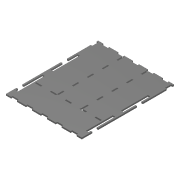
# Autodesk Inventor part: base
Saved by Autodesk Inventor 2020 (Build 240168000, 168)
## iProperties
Created: 2021-09-21
Part Number: base
Material: Generic
Document SubType Name: Modeling
Designer: pablo
Density: 1 g/cm^3
Appearance: Smooth - Black
Mass: 365.55 g
Surface Area: 1587.23 cm^2
Volume: 365.55 cm^3
Author: pablo
Autodesk Inventor part; units mm, degrees
ref_plane "YZ Plane" through (0, 0, 0) normal (1, 0, 0) x (0, 1, 0)
ref_plane "XZ Plane" through (0, 0, 0) normal (0, 1, 0) x (-1, 0, 0)
ref_plane "XY Plane" through (0, 0, 0) normal (0, 0, 1) x (1, 0, 0)
sketch "Sketch1" plane through (0, 0, 0) normal (0, 1, 0) x (-1, 0, 0)
  line L0 (127.5, -155) -> (-127.5, -155)
  line L1 (-127.5, -155) -> (-127.5, 155)
  line L2 (-127.5, 155) -> (127.5, 155)
  line L3 (127.5, 155) -> (127.5, -155)
  line L4 (127.5, -155) -> (-127.5, 155) construction
  line L5 (-127.5, -155) -> (127.5, 155) construction
  point P0 (0, 0)
  dimension "d0" = 255
  dimension "d1" = 310
  constraints: 12 end point, 2 midpoint, 2 parallel, 1 horizontal, 1 perpendicular
  measures "d0" distance of L1.end L2.end
  measures "d1" distance of L0.end L1.end
extrude "base" add sketch "Sketch1" along normal blind 5
sketch "Sketch3" plane through (0, 5, 0) normal (0, 1, 0) x (1, 0, 0)
  line L0 (127.5, 155) -> (-127.5, 155)
  line L1 (-127.5, 155) -> (-127.5, -155)
  line L2 (-127.5, 150) -> (-122.5, 150)
  line L3 (-122.5, 150) -> (-122.5, 130)
  line L4 (-122.5, 130) -> (-127.5, 130)
  line L5 (-127.5, 130) -> (-127.5, 150)
  line L6 (-127.5, 100) -> (-122.5, 100)
  line L7 (-122.5, 100) -> (-122.5, 80)
  line L8 (-122.5, 80) -> (-127.5, 80)
  line L9 (-127.5, 80) -> (-127.5, 100)
  line L10 (-127.5, 50) -> (-122.5, 50)
  line L11 (-122.5, 50) -> (-122.5, 30)
  line L12 (-122.5, 30) -> (-127.5, 30)
  line L13 (-127.5, 30) -> (-127.5, 50)
  line L14 (-127.5, 0) -> (-122.5, 0)
  line L15 (-122.5, 0) -> (-122.5, -20)
  line L16 (-122.5, -20) -> (-127.5, -20)
  line L17 (-127.5, -20) -> (-127.5, 0)
  line L18 (-127.5, -50) -> (-122.5, -50)
  line L19 (-122.5, -50) -> (-122.5, -70)
  line L20 (-122.5, -70) -> (-127.5, -70)
  line L21 (-127.5, -70) -> (-127.5, -50)
  line L22 (-127.5, -100) -> (-122.5, -100)
  line L23 (-122.5, -100) -> (-122.5, -120)
  line L24 (-122.5, -120) -> (-127.5, -120)
  line L25 (-127.5, -120) -> (-127.5, -100)
  line L26 (122.5, 50) -> (127.5, 50)
  line L27 (127.5, 30) -> (122.5, 30)
  line L28 (127.5, 50) -> (127.5, 30)
  line L29 (122.5, 30) -> (122.5, 50)
  line L30 (122.5, 0) -> (127.5, 0)
  line L31 (127.5, 0) -> (127.5, -20)
  line L32 (127.5, -20) -> (122.5, -20)
  line L33 (122.5, -20) -> (122.5, 0)
  line L34 (122.5, -50) -> (127.5, -50)
  line L35 (127.5, -50) -> (127.5, -70)
  line L36 (127.5, -70) -> (122.5, -70)
  line L37 (122.5, -70) -> (122.5, -50)
  line L38 (122.5, -100) -> (127.5, -100)
  line L39 (127.5, -100) -> (127.5, -120)
  line L40 (127.5, -120) -> (122.5, -120)
  line L41 (122.5, -120) -> (122.5, -100)
  line L42 (127.5, 80) -> (122.5, 80)
  line L43 (127.5, 100) -> (127.5, 80)
  line L44 (122.5, 80) -> (122.5, 100)
  line L45 (122.5, 100) -> (127.5, 100)
  line L46 (127.5, 130) -> (122.5, 130)
  line L47 (127.5, 150) -> (127.5, 130)
  line L48 (122.5, 130) -> (122.5, 150)
  line L49 (122.5, 150) -> (127.5, 150)
  point P0 (0, 0)
  point P1 (-127.5, 105)
  point P2 (-127.5, 55)
  point P3 (-127.5, 5)
  point P4 (-127.5, -45)
  point P5 (-127.5, -95)
  point P6 (122.5, 155)
  point P7 (122.5, 55)
  point P8 (122.5, 5)
  point P9 (122.5, -95)
  point P10 (122.5, -45)
  point P11 (122.5, 105)
  dimension "d4" = 5
  dimension "d5" = 20
  dimension "d8" = 50
  dimension "d15" = 250
  constraints: 100 end point, 1 horizontal, 1 point on line, 1 vertical, 99 other
  measures "d4" distance of L3.end L4.end
  measures "d5" distance of L2.end L3.end
  measures "d8" distance of L0.end point (-127.5, 105)
  measures "d15" distance of L0.end point (122.5, 155)
extrude "Encaixe Laterais" cut sketch "Sketch3" against normal blind 5 contours L2 L3 L4 L1 | L22 L23 L24 L1 | L10 L11 L12 L1 | L26 L28 L27 L29 | L38 L39 L40 L41 | L46 L48 L49 L47
sketch "Sketch4" plane through (0, 5, 0) normal (0, 1, 0) x (1, 0, 0)
  line L0 (-127.5, 150) -> (-122.5, 150) projected
  line L1 (122.5, 150) -> (127.5, 150) projected
  line L2 (-122.5, 150) -> (122.5, 150)
  line L3 (-40.8333, 150) -> (-35.8333, 150)
  line L4 (-35.8333, 150) -> (-35.8333, 130)
  line L5 (-35.8333, 130) -> (-40.8333, 130)
  line L6 (-40.8333, 130) -> (-40.8333, 150)
  line L7 (40.8333, 150) -> (45.8333, 150)
  line L8 (45.8333, 150) -> (45.8333, 130)
  line L9 (45.8333, 130) -> (40.8333, 130)
  line L10 (40.8333, 130) -> (40.8333, 150)
  line L11 (-40.8333, 100) -> (-35.8333, 100)
  line L12 (-35.8333, 100) -> (-35.8333, 80)
  line L13 (-35.8333, 80) -> (-40.8333, 80)
  line L14 (-40.8333, 80) -> (-40.8333, 100)
  line L15 (40.8333, 100) -> (45.8333, 100)
  line L16 (45.8333, 100) -> (45.8333, 80)
  line L17 (45.8333, 80) -> (40.8333, 80)
  line L18 (40.8333, 80) -> (40.8333, 100)
  line L19 (-40.8333, 50) -> (-35.8333, 50)
  line L20 (-35.8333, 50) -> (-35.8333, 30)
  line L21 (-35.8333, 30) -> (-40.8333, 30)
  line L22 (-40.8333, 30) -> (-40.8333, 50)
  line L23 (40.8333, 50) -> (45.8333, 50)
  line L24 (45.8333, 50) -> (45.8333, 30)
  line L25 (45.8333, 30) -> (40.8333, 30)
  line L26 (40.8333, 30) -> (40.8333, 50)
  line L27 (-40.8333, 0) -> (-35.8333, 0)
  line L28 (-35.8333, 0) -> (-35.8333, -20)
  line L29 (-35.8333, -20) -> (-40.8333, -20)
  line L30 (-40.8333, -20) -> (-40.8333, 0)
  line L31 (40.8333, 0) -> (45.8333, 0)
  line L32 (45.8333, 0) -> (45.8333, -20)
  line L33 (45.8333, -20) -> (40.8333, -20)
  line L34 (40.8333, -20) -> (40.8333, 0)
  line L35 (-40.8333, -50) -> (-35.8333, -50)
  line L36 (-35.8333, -50) -> (-35.8333, -70)
  line L37 (-35.8333, -70) -> (-40.8333, -70)
  line L38 (-40.8333, -70) -> (-40.8333, -50)
  line L39 (40.8333, -50) -> (45.8333, -50)
  line L40 (45.8333, -50) -> (45.8333, -70)
  line L41 (45.8333, -70) -> (40.8333, -70)
  line L42 (40.8333, -70) -> (40.8333, -50)
  point P0 (0, 0)
  dimension "d22" = 245
  dimension "d23" = 5
  dimension "d24" = 20
  dimension "d25" = 81.6667
  dimension "d28" = 81.6667
  dimension "d31" = 50
  constraints: 82 end point, 3 horizontal, 2 collinear, 2 parallel, 1 perpendicular, 1 point on line, 1 vertical, 70 other
  measures "d22" distance of L0.end L1.start
  measures "d23" distance of L4.end L5.end
  measures "d24" distance of L3.end L4.end
  measures "d25" distance of L0.end L3.start
  measures "d28" distance of L3.start L7.start
  measures "d31" distance of L3.start L11.start
extrude "Encaixe Divisórias 22cm" cut sketch "Sketch4" against normal blind 5
sketch "Sketch5" plane through (0, 5, 0) normal (0, 1, 0) x (1, 0, 0)
  line L0 (-127.5, -155) -> (127.5, -155) projected
  line L1 (-110, -155) -> (-90, -155)
  line L2 (-90, -155) -> (-90, -150)
  line L3 (-90, -150) -> (-110, -150)
  line L4 (-110, -150) -> (-110, -155)
  line L5 (-60, -155) -> (-40, -155)
  line L6 (-40, -155) -> (-40, -150)
  line L7 (-40, -150) -> (-60, -150)
  line L8 (-60, -150) -> (-60, -155)
  line L9 (-10, -155) -> (10, -155)
  line L10 (10, -155) -> (10, -150)
  line L11 (10, -150) -> (-10, -150)
  line L12 (-10, -150) -> (-10, -155)
  line L13 (40, -155) -> (60, -155)
  line L14 (60, -155) -> (60, -150)
  line L15 (60, -150) -> (40, -150)
  line L16 (40, -150) -> (40, -155)
  line L17 (90, -155) -> (110, -155)
  line L18 (110, -155) -> (110, -150)
  line L19 (110, -150) -> (90, -150)
  line L20 (90, -150) -> (90, -155)
  line L21 (-110, 155) -> (-110, 150)
  line L22 (-90, 155) -> (-110, 155)
  line L23 (-110, 150) -> (-90, 150)
  line L24 (-90, 150) -> (-90, 155)
  line L25 (-60, 155) -> (-60, 150)
  line L26 (-40, 155) -> (-60, 155)
  line L27 (-40, 150) -> (-40, 155)
  line L28 (-10, 155) -> (-10, 150)
  line L29 (10, 155) -> (-10, 155)
  line L30 (10, 150) -> (10, 155)
  line L31 (-10, 150) -> (10, 150)
  line L32 (-60, 150) -> (-40, 150)
  line L33 (40, 155) -> (40, 150)
  line L34 (40, 150) -> (60, 150)
  line L35 (60, 155) -> (40, 155)
  line L36 (60, 150) -> (60, 155)
  line L37 (90, 155) -> (90, 150)
  line L38 (90, 150) -> (110, 150)
  line L39 (110, 155) -> (90, 155)
  line L40 (110, 150) -> (110, 155)
  point P0 (0, 0)
  dimension "d36" = 20
  dimension "d37" = 5
  dimension "d40" = 50
  dimension "d45" = 17.5
  dimension "d46" = 17.5
  dimension "d49" = 305
  constraints: 80 end point, 2 horizontal, 2 parallel, 1 collinear, 1 perpendicular, 1 point on line, 1 vertical, 71 other
  measures "d36" distance of L3.end L2.end
  measures "d37" distance of L2.end L1.end
  measures "d40" distance of L1.start L5.start
  measures "d45" distance of L0.start L1.start
  measures "d46" distance of L17.end L0.end
  measures "d49" distance of L1.start L21.end
extrude "Extrusion4" cut sketch "Sketch5" against normal blind 5
sketch "Sketch6" plane through (0, 5, 0) normal (0, 1, 0) x (1, 0, 0)
  line L0 (-110, -155) -> (-110, -150) projected
  line L1 (110, -150) -> (110, -155) projected
  line L2 (-35.8333, -70) -> (-40.8333, -70) projected
  line L3 (-110, -70) -> (-90, -70)
  line L4 (-90, -70) -> (-90, -75)
  line L5 (-90, -75) -> (-110, -75)
  line L6 (-110, -75) -> (-110, -70)
  line L7 (-60, -70) -> (-40, -70)
  line L8 (-40, -70) -> (-40, -75)
  line L9 (-40, -75) -> (-60, -75)
  line L10 (-60, -75) -> (-60, -70)
  line L11 (-10, -70) -> (10, -70)
  line L12 (10, -70) -> (10, -75)
  line L13 (10, -75) -> (-10, -75)
  line L14 (-10, -75) -> (-10, -70)
  line L15 (40, -70) -> (60, -70)
  line L16 (60, -70) -> (60, -75)
  line L17 (60, -75) -> (40, -75)
  line L18 (40, -75) -> (40, -70)
  line L19 (90, -70) -> (110, -70)
  line L20 (110, -70) -> (110, -75)
  line L21 (110, -75) -> (90, -75)
  line L22 (90, -75) -> (90, -70)
  point P0 (0, 0)
  dimension "d56" = 20
  dimension "d57" = 5
  dimension "d60" = 50
  constraints: 40 end point, 2 horizontal, 2 parallel, 1 collinear, 1 perpendicular, 31 other
  measures "d56" distance of L4.end L5.end
  measures "d57" distance of L3.end L4.end
  measures "d60" distance of L3.start L7.start
extrude "Extrusion5" cut sketch "Sketch6" against normal blind 5
sketch "Sketch7" plane through (0, 5, 0) normal (0, 1, 0) x (1, 0, 0)
  line L0 (-127.5, -155) -> (-110, -155) projected
  line L1 (-90, -155) -> (-60, -155) projected
  line L2 (-114.5, -10) -> (-122.5, -10)
  line L3 (-122.5, -10) -> (-122.5, 80)
  line L4 (-122.5, 80) -> (-114.5, 80)
  line L5 (-114.5, 80) -> (-114.5, -10)
  line L6 (-114.5, -10) -> (-122.5, 80) construction
  line L7 (-122.5, -10) -> (-114.5, 80) construction
  line L8 (-127.5, 155) -> (-127.5, 150) projected
  line L9 (-122.5, -128) -> (-114.5, -128)
  line L10 (-114.5, -128) -> (-114.5, -38)
  line L11 (-114.5, -38) -> (-122.5, -38)
  line L12 (-122.5, -38) -> (-122.5, -128)
  line L13 (-122.5, -128) -> (-114.5, -38) construction
  line L14 (-114.5, -128) -> (-122.5, -38) construction
  line L15 (0, -20) -> (0, -40)
  line L16 (114.5, -10) -> (122.5, -10)
  line L17 (122.5, -10) -> (122.5, 80)
  line L18 (122.5, 80) -> (114.5, 80)
  line L19 (114.5, 80) -> (114.5, -10)
  line L20 (114.5, -10) -> (122.5, 80) construction
  line L21 (122.5, -10) -> (114.5, 80) construction
  line L22 (127.5, -20) -> (127.5, -50)
  line L23 (122.5, -128) -> (114.5, -128)
  line L24 (114.5, -128) -> (114.5, -38)
  line L25 (114.5, -38) -> (122.5, -38)
  line L26 (122.5, -38) -> (122.5, -128)
  line L27 (122.5, -128) -> (114.5, -38) construction
  line L28 (114.5, -128) -> (122.5, -38) construction
  point P0 (0, 0)
  point P1 (-118.5, 35)
  point P2 (-127.5, -20)
  point P3 (-127.5, -50)
  point P4 (-118.5, -83)
  point P5 (118.5, 35)
  point P6 (118.5, -83)
  dimension "d67" = 8
  dimension "d68" = 90
  dimension "d69" = 5
  dimension "d71" = 8
  dimension "d72" = 90
  dimension "d78" = 5
  dimension "d79" = 27
  dimension "d80" = 145
  constraints: 52 end point, 12 symmetric about line, 8 midpoint, 4 parallel, 2 horizontal, 2 perpendicular, 1 vertical
  measures "d67" distance of L3.end L4.end
  measures "d68" distance of L2.end L3.end
  measures "d69" distance from line of L8 L2.end
  measures "d71" distance of L11.end L10.end
  measures "d72" distance of L10.end L9.end
  measures "d78" horizontal distance of L0.start L9.start
  measures "d79" vertical distance of L0.start L9.start
  measures "d80" vertical distance of L0.start L2.end
extrude "Extrusion6" cut sketch "Sketch7" against normal blind 5
body "Solid1"
